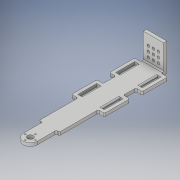
# Autodesk Inventor part: hand
Saved by Autodesk Inventor 2019 (Build 230136000, 136)
## iProperties
Created: 2018-10-22
Part Number: hand
Material: 일반
Document SubType Name: Modeling
Designer: otm09
Density: 1 g/cm^3
Appearance: 기본값
Author: otm09
Autodesk Inventor part; units mm, degrees
ref_plane "YZ Plane" through (0, 0, 0) normal (1, 0, 0) x (0, 1, 0)
ref_plane "XZ Plane" through (0, 0, 0) normal (0, 1, 0) x (-1, 0, 0)
ref_plane "XY Plane" through (0, 0, 0) normal (0, 0, 1) x (1, 0, 0)
sketch "스케치1" plane through (0, 0, 0) normal (0, 1, 0) x (-1, 0, 0)
  line L0 (32, 103.3333) -> (32, 63.3333)
  line L1 (32, 146.6667) -> (32, 106.6667)
  line L2 (0, 103.3333) -> (0, 63.3333)
  line L3 (0, 146.6667) -> (0, 106.6667)
  line L4 (0, 0) -> (32, 0)
  circle A0 centre (16, 200) radius 11
  circle A1 centre (16, 192) radius 1.1
  circle A2 centre (16, 200) radius 11
  circle A3 centre (24, 200) radius 1.1
  circle A4 centre (16, 200) radius 11
  circle A5 centre (16, 208) radius 1.1
  circle A6 centre (16, 200) radius 11
  circle A7 centre (8, 200) radius 1.1
  arc A8 (17.1384, 189.0591) -> (17.1564, 189.061) centre (16, 200) ccw
  circle A9 centre (16, 200) radius 4.5
  line L5 (27, 200) -> (27, 170)
  line L6 (27, 170) -> (32, 170)
  line L7 (32, 170) -> (32, 0)
  line L8 (5, 200) -> (5, 170)
  line L9 (5, 170) -> (0, 170)
  line L10 (0, 0) -> (0, 170)
  arc A10 (5, 200) -> (27, 200) centre (16, 200) ccw
  line L11 (0, 13.7551) -> (-5, 13.7551)
  line L12 (-5, 13.7551) -> (-5, 43.7551)
  line L13 (-5, 43.7551) -> (0, 43.7551)
  line L14 (0, 43.7551) -> (0, 13.7551)
  line L15 (32, 13.7551) -> (37, 13.7551)
  line L16 (37, 13.7551) -> (37, 43.7551)
  line L17 (37, 43.7551) -> (32, 43.7551)
  line L18 (32, 43.7551) -> (32, 13.7551)
  line L19 (32, 8.7551) -> (42, 8.7551)
  line L20 (42, 8.7551) -> (42, 48.7551)
  line L21 (42, 48.7551) -> (32, 48.7551)
  line L22 (32, 48.7551) -> (32, 8.7551)
  line L23 (0, 8.7551) -> (-10, 8.7551)
  line L24 (-10, 8.7551) -> (-10, 48.7551)
  line L25 (-10, 48.7551) -> (0, 48.7551)
  line L26 (0, 48.7551) -> (0, 8.7551)
  line L27 (0, 103.7551) -> (0, 73.7551)
  line L28 (-5, 73.7551) -> (-5, 103.7551)
  line L29 (-5, 103.7551) -> (0, 103.7551)
  line L30 (-10, 108.7551) -> (0, 108.7551)
  line L31 (0, 108.7551) -> (0, 68.7551)
  line L32 (-10, 68.7551) -> (-10, 108.7551)
  line L33 (0, 68.7551) -> (-10, 68.7551)
  line L34 (0, 73.7551) -> (-5, 73.7551)
  line L35 (42, 108.7551) -> (32, 108.7551)
  line L36 (37, 103.7551) -> (32, 103.7551)
  line L37 (32, 103.7551) -> (32, 73.7551)
  line L38 (37, 73.7551) -> (37, 103.7551)
  line L39 (32, 108.7551) -> (32, 68.7551)
  line L40 (42, 68.7551) -> (42, 108.7551)
  line L41 (32, 68.7551) -> (42, 68.7551)
  line L42 (32, 73.7551) -> (37, 73.7551)
  point P0 (32, 123.3333)
  point P1 (0, 123.3333)
  dimension "d162" = 2.2
  dimension "d163" = 360
  dimension "d164" = 9
  dimension "d165" = 30
  dimension "d166" = 5
  dimension "d167" = 30
  dimension "d170" = 5
  dimension "d171" = 30
  dimension "d174" = 5
  dimension "d175" = 5
  dimension "d176" = 5
  dimension "d177" = 5
  dimension "d180" = 60
  constraints: 86 end point, 11 centre point, 10 tangent, 9 parallel, 8 point on line, 7 point on circle, 4 horizontal, 4 perpendicular, 3 coincident, 1 vertical, 51 other
  measures "d162" diameter of A1
  measures "d164" diameter of A9
  measures "d165" distance of L5.start L5.end
  measures "d166" distance of L12.end L13.end
  measures "d167" distance of L11.end L12.end
  measures "d170" distance of L17.end L16.end
  measures "d171" distance of L16.end L15.end
  measures "d174" distance between parallel lines of L15 L19
  measures "d175" distance between parallel lines of L21 L17
  measures "d176" distance between parallel lines of L20 L16
  measures "d177" distance between parallel lines of L12 L24
  measures "d180" distance of L13.end L27.start
extrude "돌출5" add sketch "스케치1" along normal blind 5 contours L0 L7 L4 L10 L2 L3 L9 L8 A0 L5 L6 L1 | L42 L38 L36 L7 L1 L35 L40 L41 L0 | L21 L20 L19 L7 L15 L16 L17 | A0 | L23 L24 L25 L10 L13 L12 L11 | L3 L10 L29 L28 L34 L2 L33 L32 L30
sketch "스케치11" plane through (0, 5, 0) normal (0, 1, 0) x (1, 0, 0)
  line L0 (0, 0) -> (-32, 0) projected
  line L1 (0, -200) -> (0, 0) projected
  line L2 (-32, 0) -> (0, 0)
  line L3 (0, 0) -> (0, -5)
  line L4 (0, -5) -> (-32, -5)
  line L5 (-32, -5) -> (-32, 0)
  point P0 (0, -60)
  dimension "d138" = 5
  constraints: 8 end point, 2 parallel, 1 horizontal, 1 perpendicular, 1 point on line
  measures "d138" distance of L2.end L3.end
extrude "돌출11" add sketch "스케치11" along normal blind 40
sketch "스케치12" plane through (-32, 5, 5) normal (0, 0, 1) x (1, 0, 0)
  circle A0 centre (8, 24) radius 1.1
  circle A1 centre (8, 24) radius 2.1
  line L0 (32, 0) -> (0, 0) projected
  line L1 (32, 0) -> (32, 40) projected
  line L2 (0, 40) -> (32, 40) projected
  line L3 (0, 0) -> (0, 40) projected
  circle A2 centre (16, 24) radius 1.1
  circle A3 centre (16, 24) radius 2.1
  circle A4 centre (24, 24) radius 1.1
  circle A5 centre (24, 24) radius 2.1
  circle A6 centre (8, 16) radius 1.1
  circle A7 centre (8, 16) radius 2.1
  circle A8 centre (16, 16) radius 1.1
  circle A9 centre (16, 16) radius 2.1
  circle A10 centre (24, 16) radius 1.1
  circle A11 centre (24, 16) radius 2.1
  circle A12 centre (8, 8) radius 1.1
  circle A13 centre (8, 8) radius 2.1
  circle A14 centre (16, 8) radius 1.1
  circle A15 centre (16, 8) radius 2.1
  circle A16 centre (24, 8) radius 1.1
  circle A17 centre (24, 8) radius 2.1
  point P0 (32, -5)
  dimension "d141" = 2.2
  dimension "d142" = 4.2
  dimension "d145" = 8
  dimension "d148" = 8
  dimension "d151" = 16
  dimension "d152" = 16
  constraints: 18 centre point, 9 coincident, 1 horizontal, 1 vertical, 32 other
  measures "d141" diameter of A0
  measures "d142" diameter of A1
  measures "d145" distance of A0.centre A2.centre
  measures "d148" distance of A0.centre A6.centre
  measures "d151" distance from line of L1 A8.centre
  measures "d152" distance from line of L0 A8.centre
extrude "돌출12" cut sketch "스케치12" against normal blind 3 contours A0 | A1 | A2 | A3 | A4 | A5 | A6 | A7 | A8 | A9 | A10 | A11 | A12 | A13 | A14 | A15 | A16 | A17
extrude "돌출13" cut sketch "스케치12" against normal blind 5 contours A0 | A2 | A4 | A6 | A8 | A10 | A12 | A14 | A16
fillet "모깎기5" radius 2 30 edges at (-5, 2.5, 170) (0, 2.5, 170) (0, 2.5, 108.7551) (10, 2.5, 108.7551) (10, 2.5, 68.7551) (10, 2.5, 48.7551) (0, 2.5, 48.7551) (10, 2.5, 8.7551) (0, 5, 88.7551) (-32, 5, 88.7551) (-42, 2.5, 108.7551) (-32, 2.5, 170) (-42, 2.5, 48.7551) (-32, 5, 28.7551) (-42, 2.5, 8.7551) (-42, 2.5, 68.7551) (0, 5, 28.7551) (0, 2.5, 8.7551) (-32, 2.5, 8.7551) (-32, 0, 28.7551) (-32, 0, 88.7551) (0, 2.5, 68.7551) (-32, 2.5, 68.7551) (-32, 2.5, 48.7551) (-32, 2.5, 108.7551) (-27, 2.5, 170) (0, 0, 88.7551) (0, 0, 28.7551) (-16, 0, 0) (-16, 5, 5)
sketch "스케치14" plane through (0, 0, 0) normal (0, -1, 0) x (1, 0, 0)
  circle A0 centre (-24, 200) radius 1.1 projected
  circle A1 centre (-24, 200) radius 2.1
  circle A2 centre (-16, 208) radius 1.1 projected
  circle A3 centre (-16, 208) radius 2.1
  circle A4 centre (-16, 192) radius 1.1 projected
  circle A5 centre (-16, 192) radius 2.1
  circle A6 centre (-8, 200) radius 1.1 projected
  circle A7 centre (-8, 200) radius 2.1
  point P0 (0, 0)
  dimension "d192" = 4.2
  dimension "d193" = 4.2
  dimension "d194" = 4.2
  dimension "d195" = 4.2
  constraints: 4 centre point, 4 coincident
  measures "d192" diameter of A1
  measures "d193" diameter of A3
  measures "d194" diameter of A5
  measures "d195" diameter of A7
extrude "돌출15" cut sketch "스케치14" against normal blind 3
